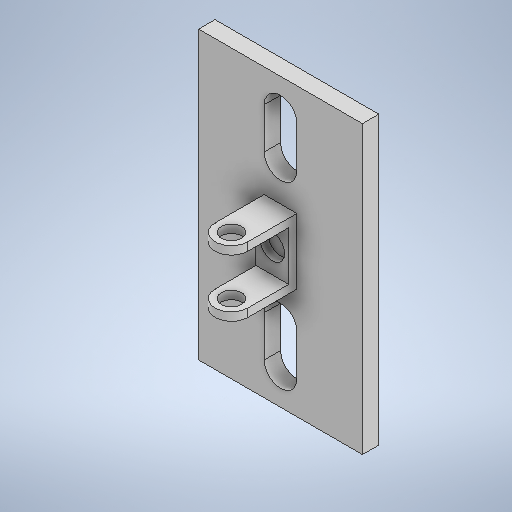
# Autodesk Inventor part: soporte_polea
Saved by Autodesk Inventor 2026 (Build 300175050, 175E)
## iProperties
Created: 2025-07-05
Part Number: soporte_polea
Material: Genérico
Document SubType Name: Modeling
Designer: piero
Density: 1 g/cm^3
Appearance: Valor por defecto
Author: piero
Autodesk Inventor part; units mm, degrees
ref_plane "YZ Plane" through (0, 0, 0) normal (1, 0, 0) x (0, 1, 0)
ref_plane "XZ Plane" through (0, 0, 0) normal (0, 1, 0) x (-1, 0, 0)
ref_plane "XY Plane" through (0, 0, 0) normal (0, 0, 1) x (1, 0, 0)
sketch "Boceto1" plane through (0, 0, 0) normal (0, 0, 1) x (1, 0, 0)
  line L0 (0, 0) -> (20, 0)
  line L1 (20, 0) -> (20, 35)
  line L2 (20, 35) -> (0, 35)
  line L3 (0, 35) -> (0, 0)
  line L4 (10, 31) -> (10, 26) construction
  line L5 (8, 31) -> (8, 26)
  line L6 (12, 26) -> (12, 31)
  arc A0 (12, 31) -> (8, 31) centre (10, 31) ccw
  arc A1 (8, 26) -> (12, 26) centre (10, 26) ccw
  line L7 (10, 4) -> (10, 9) construction
  line L8 (12, 4) -> (12, 9)
  line L9 (8, 9) -> (8, 4)
  arc A2 (8, 4) -> (12, 4) centre (10, 4) ccw
  arc A3 (12, 9) -> (8, 9) centre (10, 9) ccw
  point P0 (10, 28.5)
  point P1 (10, 6.5)
  point P2 (10, 33)
  point P3 (10, 2)
  point P4 (10, 11)
  point P5 (10, 24)
  dimension "d0" = 20
  dimension "d1" = 35
  dimension "d2" = 5
  dimension "d3" = 4
  dimension "d4" = 5
  dimension "d5" = 4
  dimension "d6" = 2
  dimension "d7" = 2
  dimension "d8" = 13
  constraints: 24 end point, 12 point on circle, 8 tangent, 4 centre point, 4 parallel, 2 midpoint, 2 point on line, 1 horizontal, 1 perpendicular, 1 vertical
  measures "d0" distance of L2.end L1.end
  measures "d1" distance of L1.end L0.end
  measures "d2" distance of L4.start L4.end
  measures "d3" diameter of A1
  measures "d4" distance of L7.start L7.end
  measures "d5" diameter of A3
  measures "d6" distance from line of point (10, 33) L2
  measures "d7" distance from line of point (10, 2) L0
  measures "d8" distance of point (10, 11) point (10, 24)
extrude "Extrusión1" add sketch "Boceto1" along normal blind 2
sketch "Boceto2" plane through (0, 0, 2) normal (0, 0, 1) x (1, 0, 0)
  line L0 (8, 26) -> (8, 31) projected
  line L1 (12, 31) -> (12, 26) projected
  line L2 (8, 21.5) -> (12, 21.5)
  line L3 (12, 21.5) -> (12, 13.5)
  line L4 (12, 13.5) -> (8, 13.5)
  line L5 (8, 13.5) -> (8, 21.5)
  arc A0 (8, 26) -> (12, 26) centre (10, 26) ccw projected
  arc A1 (12, 9) -> (8, 9) centre (10, 9) ccw projected
  circle A2 centre (10, 17.5) radius 1.5
  point P0 (0, 0)
  point P1 (10, 21.5)
  point P2 (10, 24)
  point P3 (10, 13.5)
  point P4 (10, 11)
  dimension "d11" = 4
  dimension "d12" = 8
  dimension "d13" = 2.5
  dimension "d15" = 3
  constraints: 8 end point, 2 midpoint, 2 parallel, 2 point on circle, 1 centre point, 1 horizontal, 1 perpendicular
  measures "d11" distance of L3.end L4.end
  measures "d12" distance of L2.end L3.end
  measures "d13" distance of point (10, 21.5) point (10, 24)
  measures "d15" diameter of A2
extrude "Extrusión2" add sketch "Boceto2" along normal blind 1
sketch "Boceto3" plane through (8, 21.5, 2) normal (0, 1, 0) x (1, 0, 0)
  line L0 (0, -1) -> (0, -6)
  line L1 (4, -1) -> (4, -6)
  arc A0 (0, -6) -> (4, -6) centre (2, -6) ccw
  circle A1 centre (2, -6) radius 1.25
  line L2 (0, -1) -> (4, -1) projected
  line L3 (0, -1) -> (4, -1)
  point P0 (-8, 2)
  dimension "d18" = 5
  dimension "d19" = 5
  dimension "d20" = 2
  dimension "d21" = 2.5
  constraints: 6 end point, 2 centre point, 2 point on circle, 2 vertical, 1 coincident, 1 collinear
  measures "d18" distance of L0.start L0.end
  measures "d19" distance of L1.start L1.end
  measures "d20" radius of A0
  measures "d21" diameter of A1
extrude "Extrusión3" add sketch "Boceto3" against normal blind 1
sketch "Boceto4" plane through (8, 13.5, 2) normal (0, -1, 0) x (1, 0, 0)
  line L0 (0, 0) -> (0, 6) projected
  line L1 (0, 1) -> (0, 6)
  line L2 (4, 0) -> (4, 1) projected
  line L3 (4, 1) -> (4, 6) projected
  line L4 (4, 1) -> (4, 6)
  arc A0 (4, 6) -> (0, 6) centre (2, 6) ccw
  circle A1 centre (2, 6) radius 1.25
  line L5 (0, 1) -> (4, 1) projected
  line L6 (0, 1) -> (4, 1)
  point P0 (-8, -2)
  dimension "d25" = 2.5
  constraints: 6 end point, 2 centre point, 2 point on circle, 2 tangent, 1 coincident, 1 collinear, 1 perpendicular, 1 vertical
  measures "d25" diameter of A1
extrude "Extrusión4" add sketch "Boceto4" against normal blind 1
